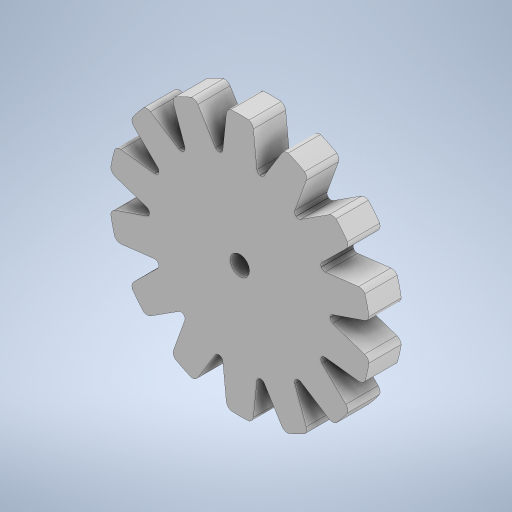
# Autodesk Inventor part: Zebatka
Saved by Autodesk Inventor 2024 (Build 280153000, 153)
## iProperties
Created: 2025-05-18
Part Number: Zebatka
Material: Ogólny
Document SubType Name: Modeling
Designer: Victoria
Density: 1 g/cm^3
Appearance: Domyślna
Author: Victoria
Autodesk Inventor part; units mm, degrees
ref_plane "YZ Plane" through (0, 0, 0) normal (1, 0, 0) x (0, 1, 0)
ref_plane "XZ Plane" through (0, 0, 0) normal (0, 1, 0) x (-1, 0, 0)
ref_plane "XY Plane" through (0, 0, 0) normal (0, 0, 1) x (1, 0, 0)
sketch "Szkic2" plane through (0, 0, 0) normal (0, 0, 1) x (1, 0, 0)
  circle A0 centre (0, 0) radius 20.25
  line L0 (0, 20.25) -> (1.0996, 20.25)
  line L1 (0, 20.25) -> (-1.0996, 20.25)
  circle A1 centre (0, 0) radius 14
  line L2 (-2.0941, 19.3545) -> (-2.6842, 13.7403)
  line L3 (-2, 20.25) -> (3.6452, 20.25) construction
  line L4 (2.0941, 19.3545) -> (2.6842, 13.7403)
  line L5 (2, 20.25) -> (7.6452, 20.25) construction
  arc A2 (-1.0996, 20.25) -> (-2.0941, 19.3545) centre (-1.0996, 19.25) ccw
  arc A3 (2.0941, 19.3545) -> (1.0996, 20.25) centre (1.0996, 19.25) ccw
  line L6 (-10.2844, 16.5292) -> (-8.3801, 11.2149)
  arc A4 (-9.7768, 17.7675) -> (-10.2844, 16.5292) centre (-9.343, 16.8666) ccw
  line L7 (-8.7861, 18.2446) -> (-9.7768, 17.7675)
  line L8 (-8.7861, 18.2446) -> (-7.7954, 18.7217)
  arc A5 (-6.5109, 18.3464) -> (-7.7954, 18.7217) centre (-7.3616, 17.8207) ccw
  line L9 (-6.5109, 18.3464) -> (-3.5433, 13.5442)
  line L10 (-16.4376, 10.4301) -> (-12.4161, 6.4683)
  arc A6 (-16.5177, 11.766) -> (-16.4376, 10.4301) centre (-15.7358, 11.1425) ccw
  line L11 (-15.8321, 12.6257) -> (-16.5177, 11.766)
  line L12 (-15.8321, 12.6257) -> (-15.1465, 13.4854)
  arc A7 (-13.8263, 13.7046) -> (-15.1465, 13.4854) centre (-14.3647, 12.8619) ccw
  line L13 (-13.8263, 13.7046) -> (-9.069, 10.6655)
  line L14 (-19.3353, 2.2652) -> (-13.9931, 0.4406)
  arc A8 (-19.987, 3.434) -> (-19.3353, 2.2652) centre (-19.012, 3.2115) ccw
  line L15 (-19.7423, 4.506) -> (-19.987, 3.434)
  line L16 (-19.7423, 4.506) -> (-19.4976, 5.5781)
  arc A9 (-18.4033, 6.3484) -> (-19.4976, 5.5781) centre (-18.5227, 5.3556) ccw
  line L17 (-18.4033, 6.3484) -> (-12.7985, 5.6744)
  line L18 (-18.4033, -6.3484) -> (-12.7985, -5.6744)
  arc A10 (-19.4976, -5.5781) -> (-18.4033, -6.3484) centre (-18.5227, -5.3556) ccw
  line L19 (-19.7423, -4.506) -> (-19.4976, -5.5781)
  line L20 (-19.7423, -4.506) -> (-19.987, -3.434)
  arc A11 (-19.3353, -2.2652) -> (-19.987, -3.434) centre (-19.012, -3.2115) ccw
  line L21 (-19.3353, -2.2652) -> (-13.9931, -0.4406)
  line L22 (-13.8263, -13.7046) -> (-9.069, -10.6655)
  arc A12 (-15.1465, -13.4854) -> (-13.8263, -13.7046) centre (-14.3647, -12.8619) ccw
  line L23 (-15.8321, -12.6257) -> (-15.1465, -13.4854)
  line L24 (-15.8321, -12.6257) -> (-16.5177, -11.766)
  arc A13 (-16.4376, -10.4301) -> (-16.5177, -11.766) centre (-15.7358, -11.1425) ccw
  line L25 (-16.4376, -10.4301) -> (-12.4161, -6.4683)
  line L26 (-6.5109, -18.3464) -> (-3.5433, -13.5442)
  arc A14 (-7.7954, -18.7217) -> (-6.5109, -18.3464) centre (-7.3616, -17.8207) ccw
  line L27 (-8.7861, -18.2446) -> (-7.7954, -18.7217)
  line L28 (-8.7861, -18.2446) -> (-9.7768, -17.7675)
  arc A15 (-10.2844, -16.5292) -> (-9.7768, -17.7675) centre (-9.343, -16.8666) ccw
  line L29 (-10.2844, -16.5292) -> (-8.3801, -11.2149)
  line L30 (2.0941, -19.3545) -> (2.6842, -13.7403)
  arc A16 (1.0996, -20.25) -> (2.0941, -19.3545) centre (1.0996, -19.25) ccw
  line L31 (0, -20.25) -> (1.0996, -20.25)
  line L32 (0, -20.25) -> (-1.0996, -20.25)
  arc A17 (-2.0941, -19.3545) -> (-1.0996, -20.25) centre (-1.0996, -19.25) ccw
  line L33 (-2.0941, -19.3545) -> (-2.6842, -13.7403)
  line L34 (10.2844, -16.5292) -> (8.3801, -11.2149)
  arc A18 (9.7768, -17.7675) -> (10.2844, -16.5292) centre (9.343, -16.8666) ccw
  line L35 (8.7861, -18.2446) -> (9.7768, -17.7675)
  line L36 (8.7861, -18.2446) -> (7.7954, -18.7217)
  arc A19 (6.5109, -18.3464) -> (7.7954, -18.7217) centre (7.3616, -17.8207) ccw
  line L37 (6.5109, -18.3464) -> (3.5433, -13.5442)
  line L38 (16.4376, -10.4301) -> (12.4161, -6.4683)
  arc A20 (16.5177, -11.766) -> (16.4376, -10.4301) centre (15.7358, -11.1425) ccw
  line L39 (15.8321, -12.6257) -> (16.5177, -11.766)
  line L40 (15.8321, -12.6257) -> (15.1465, -13.4854)
  arc A21 (13.8263, -13.7046) -> (15.1465, -13.4854) centre (14.3647, -12.8619) ccw
  line L41 (13.8263, -13.7046) -> (9.069, -10.6655)
  line L42 (19.3353, -2.2652) -> (13.9931, -0.4406)
  arc A22 (19.987, -3.434) -> (19.3353, -2.2652) centre (19.012, -3.2115) ccw
  line L43 (19.7423, -4.506) -> (19.987, -3.434)
  line L44 (19.7423, -4.506) -> (19.4976, -5.5781)
  arc A23 (18.4033, -6.3484) -> (19.4976, -5.5781) centre (18.5227, -5.3556) ccw
  line L45 (18.4033, -6.3484) -> (12.7985, -5.6744)
  line L46 (18.4033, 6.3484) -> (12.7985, 5.6744)
  arc A24 (19.4976, 5.5781) -> (18.4033, 6.3484) centre (18.5227, 5.3556) ccw
  line L47 (19.7423, 4.506) -> (19.4976, 5.5781)
  line L48 (19.7423, 4.506) -> (19.987, 3.434)
  arc A25 (19.3353, 2.2652) -> (19.987, 3.434) centre (19.012, 3.2115) ccw
  line L49 (19.3353, 2.2652) -> (13.9931, 0.4406)
  line L50 (13.8263, 13.7046) -> (9.069, 10.6655)
  arc A26 (15.1465, 13.4854) -> (13.8263, 13.7046) centre (14.3647, 12.8619) ccw
  line L51 (15.8321, 12.6257) -> (15.1465, 13.4854)
  line L52 (15.8321, 12.6257) -> (16.5177, 11.766)
  arc A27 (16.4376, 10.4301) -> (16.5177, 11.766) centre (15.7358, 11.1425) ccw
  line L53 (16.4376, 10.4301) -> (12.4161, 6.4683)
  line L54 (6.5109, 18.3464) -> (3.5433, 13.5442)
  arc A28 (7.7954, 18.7217) -> (6.5109, 18.3464) centre (7.3616, 17.8207) ccw
  line L55 (8.7861, 18.2446) -> (7.7954, 18.7217)
  line L56 (8.7861, 18.2446) -> (9.7768, 17.7675)
  arc A29 (10.2844, 16.5292) -> (9.7768, 17.7675) centre (9.343, 16.8666) ccw
  line L57 (10.2844, 16.5292) -> (8.3801, 11.2149)
  circle A30 centre (0, 0) radius 1.5
  point P0 (-10.5881, 17.3769)
  point P1 (-6.9842, 19.1124)
  point P2 (-17.0791, 11.062)
  point P3 (-14.5851, 14.1893)
  point P4 (-20.1873, 2.5562)
  point P5 (-19.2972, 6.4559)
  point P6 (-19.2972, -6.4559)
  point P7 (-20.1873, -2.5562)
  point P8 (-14.5851, -14.1893)
  point P9 (-17.0791, -11.062)
  point P10 (-6.9842, -19.1124)
  point P11 (-10.5881, -17.3769)
  point P12 (2, -20.25)
  point P13 (-2, -20.25)
  point P14 (10.5881, -17.3769)
  point P15 (6.9842, -19.1124)
  point P16 (17.0791, -11.062)
  point P17 (14.5851, -14.1893)
  point P18 (20.1873, -2.5562)
  point P19 (19.2972, -6.4559)
  point P20 (19.2972, 6.4559)
  point P21 (20.1873, 2.5562)
  point P22 (14.5851, 14.1893)
  point P23 (17.0791, 11.062)
  point P24 (6.9842, 19.1124)
  point P25 (10.5881, 17.3769)
  point P26 (-14.9152, 13.6967)
  point P27 (-16.6722, 11.4934)
  point P28 (-19.3809, 5.8688)
  point P29 (-20.008, 3.1214)
  point P30 (-20.008, -3.1214)
  point P31 (-19.3809, -5.8688)
  point P32 (-16.6722, -11.4934)
  point P33 (-14.9152, -13.6967)
  point P34 (-10.0343, -17.589)
  point P35 (-7.4954, -18.8118)
  point P36 (-1.409, -20.2009)
  point P37 (1.409, -20.2009)
  point P38 (7.4954, -18.8118)
  point P39 (10.0343, -17.589)
  point P40 (14.9152, -13.6967)
  point P41 (16.6722, -11.4934)
  point P42 (19.3809, -5.8688)
  point P43 (20.008, -3.1214)
  point P44 (20.008, 3.1214)
  point P45 (19.3809, 5.8688)
  point P46 (16.6722, 11.4934)
  point P47 (14.9152, 13.6967)
  point P48 (10.0343, 17.589)
  point P49 (7.4954, 18.8118)
  point P50 (1.409, 20.2009)
  point P51 (-1.409, 20.2009)
  point P52 (-7.4954, 18.8118)
  point P53 (-10.0343, 17.589)
  dimension "d14" = 40.5
  dimension "d17" = 6.25
  dimension "d15" = 2
  dimension "d16" = 2
  dimension "d18" = 264
  dimension "d19" = 84
  dimension "d20" = 1
  dimension "d23" = 360
  dimension "d25" = 3
  constraints: 116 end point, 70 point on line, 56 point on circle, 29 centre point, 4 horizontal, 4 tangent, 2 coincident, 2 equal length, 1 equal radius, 246 other
  measures "d15" distance of L0.start L5.start
  measures "d16" distance of L0.start L3.start
  measures "d19" angle of L4 L5
  measures "d20" radius of A2
  measures "d25" diameter of A30
extrude "Wyciągnięcie proste2" add sketch "Szkic2" along normal blind 5 contours A25 L49 A1 L46 A24 A0 | A0 A23 L45 A1 L42 A22 | A1 | A27 L53 A1 L50 A26 A0 | A0 A21 L41 A1 L38 A20 | A29 L57 A1 L54 A28 A0 | A0 A19 L37 A1 L34 A18 | A1 L2 A2 A0 A3 L4 | L30 A16 A0 A17 L33 A1 | A1 L6 A4 A0 A5 L9 | L26 A14 A0 A15 L29 A1 | A1 L10 A6 A0 A7 L13 | L22 A12 A0 A13 L25 A1 | A1 L14 A8 A0 A9 L17 | L18 A10 A0 A11 L21 A1
fillet "Zaokrąglenie1" radius 0.6 28 edges at (-13.9931, 0.4406, 2.5) (-13.9931, -0.4406, 2.5) (-12.7985, -5.6744, 2.5) (-12.4161, -6.4683, 2.5) (-8.3801, -11.2149, 2.5) (-9.069, -10.6655, 2.5) (-2.6842, -13.7403, 2.5) (-3.5433, -13.5442, 2.5) (3.5433, -13.5442, 2.5) (2.6842, -13.7403, 2.5) (9.069, -10.6655, 2.5) (8.3801, -11.2149, 2.5) (12.7985, -5.6744, 2.5) (12.4161, -6.4683, 2.5) (13.9931, 0.4406, 2.5) (13.9931, -0.4406, 2.5) (12.7985, 5.6744, 2.5) (12.4161, 6.4683, 2.5) (8.3801, 11.2149, 2.5) (9.069, 10.6655, 2.5) (2.6842, 13.7403, 2.5) (3.5433, 13.5442, 2.5) (-3.5433, 13.5442, 2.5) (-2.6842, 13.7403, 2.5) (-9.069, 10.6655, 2.5) (-8.3801, 11.2149, 2.5) (-12.7985, 5.6744, 2.5) (-12.4161, 6.4683, 2.5)
